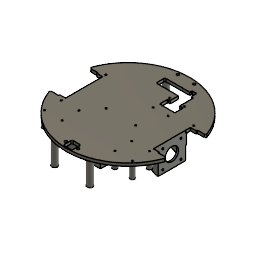
FEKTBOT_base_ver_1_2 (Autodesk Fusion 360 design; units mm, degrees)
Autodesk Fusion 360 part; units mm, degrees
note: some values were not read from the file. Set by a fixed rule: which sketch regions a step uses.
(part 1 of 2)
sketch "zakladna" plane through (0, 0, 0) normal (0, 1, 0) x (1, 0, 0)
  line L0 (-40.0372, -23.4927) -> (-85, -23.4927)
  line L1 (39.9628, -23.4927) -> (85, -23.4927)
  line L2 (-85, 23.5073) -> (-40.0372, 23.5073)
  line L3 (85, 23.5073) -> (39.9628, 23.5073)
  line L4 (1.75, 0) -> (22.5, 0)
  line L5 (-96.7123, 33.4364) -> (-85, 33.4364)
  line L6 (-85, 33.4364) -> (-85, 23.5073)
  line L7 (-96.7154, -33.4277) -> (-85, -33.4277)
  line L8 (-85, -33.4277) -> (-85, -23.4927)
  line L9 (96.7154, -33.4277) -> (85, -33.4277)
  line L10 (85, -33.4277) -> (85, -23.4927)
  line L11 (96.7123, 33.4364) -> (85, 33.4364)
  line L12 (85, 33.4364) -> (85, 23.5073)
  arc A0 (-98.5934, -36.1156) -> (98.5934, -36.1156) centre (0, 0) ccw
  arc A1 (-96.7154, -33.4277) -> (-98.5934, -36.1156) centre (-96.7154, -35.4277) ccw
  arc A2 (-98.5902, 36.1245) -> (-96.7123, 33.4364) centre (-96.7123, 35.4364) ccw
  arc A3 (96.7123, 33.4364) -> (98.5902, 36.1245) centre (96.7123, 35.4364) ccw
  arc A4 (98.5934, -36.1156) -> (96.7154, -33.4277) centre (96.7154, -35.4277) ccw
  line L13 (0, -1.75) -> (0, -22.5)
  line L14 (39.9628, -23.4927) -> (34.9628, -23.4927)
  line L15 (34.9628, -23.4927) -> (34.9628, 23.5073)
  line L16 (34.9628, 23.5073) -> (39.9628, 23.5073)
  line L17 (-40.0372, -23.4927) -> (-35.0372, -23.4927)
  line L18 (-35.0372, -23.4927) -> (-35.0372, 23.5073)
  line L19 (-35.0372, 23.5073) -> (-40.0372, 23.5073)
  line L20 (0, -20) -> (0, -2.5)
  line L21 (2.5, 0) -> (20, 0)
  line L22 (0, 105) -> (0, -105) construction
  line L23 (-105, 0) -> (104.2756, 0.0073) construction
  line L24 (-40, -12.9977) -> (44.2998, -12.9948) construction
  circle A5 centre (-25, -11.9963) radius 1.4
  circle A6 centre (-75, 37.0037) radius 1.4
  circle A7 centre (25, -11.9963) radius 1.4
  circle A8 centre (75, 37.0037) radius 1.4
  line L25 (-20, 83.0037) -> (20, 83.0037)
  line L26 (20, 83.0037) -> (20, 68.0037)
  line L27 (20, 68.0037) -> (-20, 68.0037)
  line L28 (-20, 68.0037) -> (-20, 83.0037)
  circle A9 centre (-10.5, -95.4967) radius 2.1
  circle A10 centre (10.5, -95.4967) radius 2.1
  line L29 (-5.5, -87.9967) -> (5.5, -87.9967)
  line L30 (7.5, -89.9967) -> (7.5, -100.9967)
  line L31 (5.5, -102.9967) -> (-5.5, -102.9967)
  line L32 (-7.5, -100.9967) -> (-7.5, -89.9967)
  line L33 (-10.5, -95.4967) -> (10.5, -95.4967) construction
  arc A11 (-5.5, -87.9967) -> (-7.5, -89.9967) centre (-5.5, -89.9967) ccw
  arc A12 (7.5, -89.9967) -> (5.5, -87.9967) centre (5.5, -89.9967) ccw
  arc A13 (5.5, -102.9967) -> (7.5, -100.9967) centre (5.5, -100.9967) ccw
  arc A14 (-7.5, -100.9967) -> (-5.5, -102.9967) centre (-5.5, -100.9967) ccw
  arc A15 (98.5902, 36.1245) -> (15, 103.923) centre (0, 0) ccw
  arc A16 (-15, 103.923) -> (-98.5902, 36.1245) centre (0, 0) ccw
  line L34 (75, -38.4927) -> (45, -38.4927) construction
  line L35 (45, -38.4927) -> (45, -67.4927) construction
  line L36 (45, -67.4927) -> (75, -67.4927) construction
  line L37 (75, -67.4927) -> (75, -38.4927) construction
  circle A17 centre (45, -38.4927) radius 1.375
  circle A18 centre (75, -38.4927) radius 1.375
  circle A19 centre (45, -67.4927) radius 1.375
  circle A20 centre (75, -67.4927) radius 1.375
  circle A21 centre (-45, -38.4927) radius 1.375
  circle A22 centre (-75, -38.4927) radius 1.375
  circle A23 centre (-75, -67.4927) radius 1.375
  circle A24 centre (-45, -67.4927) radius 1.375
  line L38 (34.9628, -23.4927) -> (74.9628, -23.4927)
  line L39 (74.9628, -23.4927) -> (74.9628, 23.5073)
  line L40 (74.9628, 23.5073) -> (34.9628, 23.5073)
  line L41 (34.9628, 23.5073) -> (34.9628, -23.4927)
  line L42 (-35.0372, -23.4927) -> (-75.0372, -23.4927)
  line L43 (-75.0372, -23.4927) -> (-75.0372, 23.5073)
  line L44 (-75.0372, 23.5073) -> (-35.0372, 23.5073)
  line L45 (-35.0372, 23.5073) -> (-35.0372, -23.4927)
  arc A25 (15, 103.923) -> (-15, 103.923) centre (0, 0) ccw
  line L46 (22, 99) -> (-25, 99) construction
  circle A26 centre (-14, 99) radius 2.1
  circle A27 centre (14, 99) radius 2.1
  point P0 (-82.0372, 22.8073)
  point P1 (-17.0372, -22.7927)
  point P2 (-0.0372, 0.0073)
  point P3 (81.9628, 22.8073)
  point P4 (-82.0372, -22.7927)
  point P5 (16.9628, 22.8073)
  point P6 (16.9628, 27.0073)
  point P7 (-17.0372, 27.0073)
  point P8 (81.9628, -22.7927)
  point P9 (16.9628, -22.7927)
  point P10 (16.9628, -26.9927)
  point P11 (-7.5, -87.9967)
  point P12 (7.5, -87.9967)
  point P13 (-7.5, -102.9967)
  dimension "d87" = 210
  dimension "d134" = 2
  dimension "d135" = 2
  dimension "d136" = 2
  dimension "d137" = 2
  dimension "d197" = 47
  dimension "d199" = 47
  dimension "d205" = 13
  dimension "d206" = 2.8
  dimension "d207" = 2.8
  dimension "d208" = 49
  dimension "d209" = 50
  dimension "d210" = 40
  dimension "d211" = 15
  dimension "d212" = 80
  dimension "d216" = 4.2
  dimension "d217" = 10.5
  dimension "d220" = 15
  dimension "d221" = 15
  dimension "d222" = 2
  dimension "d223" = 2
  dimension "d224" = 2
  dimension "d225" = 2
  dimension "d232" = 95.5
  dimension "d237" = 25
  dimension "d258" = 30
  dimension "d259" = 29
  dimension "d260" = 2.75
  dimension "d261" = 2.75
  dimension "d262" = 2.75
  dimension "d263" = 2.75
  dimension "d264" = 45
  dimension "d265" = 15
  dimension "d266" = 40
  dimension "d267" = 40
  dimension "d268" = 47
  dimension "d346" = 4.2
  dimension "d349" = 14
  constraint horizontal L2
  constraint horizontal L0
  constraint horizontal L3
  constraint horizontal L1
  constraint horizontal L5
  constraint vertical L6
  constraint horizontal L7
  constraint vertical L8
  constraint horizontal L9
  constraint vertical L10
  constraint horizontal L11
  constraint vertical L12
  constraint coincident A0.centre A15.centre
  constraint concentric A0 A15
  constraint tangent A0 A1
  constraint tangent L7 A1
  constraint tangent A2 A15
  constraint tangent L5 A2
  constraint tangent L11 A3
  constraint tangent A3 A15
  constraint tangent L9 A4
  constraint tangent A0 A4
  constraint horizontal L14
  constraint vertical L15
  constraint horizontal L16
  constraint horizontal L17
  constraint vertical L18
  constraint horizontal L19
  constraint midpoint A0 L22.end
  constraint parallel L20 L22
  constraint parallel L23 L24
  constraint symmetric L22 A5 A7
  constraint symmetric L22 A6 A8
  constraint horizontal L25
  constraint vertical L26
  constraint horizontal L27
  constraint vertical L28
  constraint symmetric L22 L26 L28
  constraint symmetric L22 A9 A10
  constraint horizontal L29
  constraint vertical L30
  constraint horizontal L31
  constraint vertical L32
  constraint symmetric L22 L30 L32
  constraint coincident A9.centre L33.start
  constraint coincident A10.centre L33.end
  constraint symmetric L29 L31 L33
  constraint coincident P11 L29
  constraint coincident P11 L32
  constraint tangent L29 A11
  constraint tangent L32 A11
  constraint coincident P12 L29
  constraint coincident P12 L30
  constraint tangent L29 A12
  constraint tangent L30 A12
  constraint tangent L30 A13
  constraint tangent L31 A13
  constraint coincident P13 L31
  constraint coincident P13 L32
  constraint tangent L31 A14
  constraint tangent L32 A14
  constraint concentric A15 A16
  constraint coincident L22.start A15
  constraint horizontal L34
  constraint vertical L35
  constraint horizontal L36
  constraint vertical L37
  constraint coincident L34.end L35.start
  constraint coincident L34.start L37.end
  constraint coincident L35.end L36.start
  constraint coincident L36.end L37.start
  constraint symmetric L22 A17 A21
  constraint symmetric L22 A18 A22
  constraint symmetric L22 A19 A24
  constraint symmetric L22 A20 A23
  constraint horizontal L38
  constraint vertical L39
  constraint horizontal L40
  constraint vertical L41
  constraint horizontal L42
  constraint vertical L43
  constraint horizontal L44
  constraint vertical L45
  constraint coincident L22.start A25
  constraint horizontal L46
  constraint coincident L46 A26.centre
  constraint symmetric L22 A26 A27
  measures "d87" diameter of A15
  measures "d134" radius of A1
  measures "d135" radius of A2
  measures "d136" radius of A3
  measures "d137" radius of A4
  measures "d197" distance of L1.start L3.end
  measures "d199" distance of L0.start L2.end
  measures "d205" distance of L23 L24
  measures "d206" diameter of A5
  measures "d207" diameter of A6
  measures "d208" vertical distance of A5.centre A6.centre
  measures "d209" horizontal distance of A5.centre A6.centre
  measures "d210" distance of L25.start L25.end
  measures "d211" distance of L25.start L27.end
  measures "d212" distance of A7.centre L27
  measures "d216" diameter of A9
  measures "d217" distance of L22 A9.centre
  measures "d220" distance of P11 P12
  measures "d221" distance of P11 P13
  measures "d222" radius of A11
  measures "d223" radius of A12
  measures "d224" radius of A13
  measures "d225" radius of A14
  measures "d232" distance of L23 A9.centre
  measures "d237" distance of L22 A5.centre
  measures "d258" distance of L34.start L34.end
  measures "d259" distance of L34.start L36.end
  measures "d260" diameter of A17
  measures "d261" diameter of A18
  measures "d262" diameter of A19
  measures "d263" diameter of A20
  measures "d264" distance of L22 L34.end
  measures "d265" distance of L1 L34.end
  measures "d266" distance of L14.end L38.end
  measures "d267" distance of L17.end L42.end
  measures "d268" distance of L17.end L18.end
  measures "d346" diameter of A26
  measures "d349" distance of L22 A26.centre
extrude "Extrude23" add sketch "zakladna" along normal blind 5 contours L0 L1 L2 L3 L5 L6 L7 L8 L9 L10 L11 L12 A0 A1 A2 A3 A4 L14 L15 L16 L17 L18 L19 A15 A16 L38 L40 L41 L42 L44 L45 A25 | A26 | A27
sketch "beterka" plane through (0, 0, 0) normal (0, 1, 0) x (1, 0, 0)
  line L0 (-34, -25) -> (34, -25)
  line L1 (34, -25) -> (34, -81)
  line L2 (34, -81) -> (-34, -81)
  line L3 (-34, -81) -> (-34, -25)
  line L4 (0, 105) -> (0, -105)
  line L5 (2.5, 0) -> (20, 0)
  line L6 (37.5, -84.5) -> (-37.5, -84.5)
  line L7 (-37.5, -84.5) -> (-37.5, -21.5)
  line L8 (-37.5, -21.5) -> (37.5, -21.5)
  line L9 (37.5, -21.5) -> (37.5, -84.5)
  dimension "d228" = 68
  dimension "d229" = 56
  dimension "d230" = 25
  dimension "d231" = -3.5
  constraint horizontal L0
  constraint vertical L1
  constraint horizontal L2
  constraint vertical L3
  constraint symmetric L1 L3 L4
  measures "d228" distance of L0.start L0.end
  measures "d229" distance of L0.start L2.end
  measures "d230" distance of L0 L5
extrude "Extrude25" add sketch "beterka" against normal blind 17 contours L0 L2 L3 L4 L6 L7 L8 | L0 L1 L2 L4 L6 L8 L9
sketch "zvyseni" plane through (0, 0, 0) normal (0, 1, 0) x (1, 0, 0)
  circle A0 centre (25, -11.9963) radius 4
  circle A1 centre (25, -11.9963) radius 1.4
  circle A2 centre (-25, -11.9963) radius 1.4
  circle A3 centre (-25, -11.9963) radius 4
  circle A4 centre (75, 37.0037) radius 1.4
  circle A5 centre (75, 37.0037) radius 4
  circle A6 centre (-75, 37.0037) radius 1.4
  circle A7 centre (-75, 37.0037) radius 4
  line L0 (5, 90) -> (-5, 90)
  line L1 (-5, 90) -> (-5, 85)
  line L2 (-5, 85) -> (5, 85)
  line L3 (5, 85) -> (5, 90)
  point P0 (25, -11.9963)
  point P1 (-25, -11.9963)
  point P2 (75, 37.0037)
  point P3 (-75, 37.0037)
  dimension "d250" = 8
  dimension "d251" = 8
  dimension "d252" = 8
  dimension "d253" = 8
  constraint coincident P0 A0.centre
  constraint coincident P1 A2.centre
  constraint coincident P2 A4.centre
  constraint concentric A4 A5
  constraint coincident P3 A6.centre
  constraint concentric A6 A7
  constraint horizontal L0
  constraint vertical L1
  constraint horizontal L2
  constraint vertical L3
  measures "d250" diameter of A0
  measures "d251" diameter of A3
  measures "d252" diameter of A5
  measures "d253" diameter of A7
extrude "Extrude26" add sketch "zvyseni" against normal blind 1.6
sketch " motory_podklad" plane through (0, 5, 0) normal (0, 1, 0) x (-1, 0, 0)
  circle A0 centre (-45, 67.4927) radius 1.375
  circle A1 centre (-10.5, 95.4967) radius 2.1
  circle A2 centre (-75, 38.4927) radius 1.375
  arc A3 (5.5, 87.9967) -> (7.5, 89.9967) centre (5.5, 89.9967) ccw
  line L0 (5.5, 87.9967) -> (-5.5, 87.9967)
  arc A4 (-7.5, 89.9967) -> (-5.5, 87.9967) centre (-5.5, 89.9967) ccw
  line L1 (-7.5, 89.9967) -> (-7.5, 100.9967)
  arc A5 (-5.5, 102.9967) -> (-7.5, 100.9967) centre (-5.5, 100.9967) ccw
  line L2 (-5.5, 102.9967) -> (5.5, 102.9967)
  arc A6 (7.5, 100.9967) -> (5.5, 102.9967) centre (5.5, 100.9967) ccw
  line L3 (7.5, 100.9967) -> (7.5, 89.9967)
  circle A7 centre (-75, -37.0037) radius 1.4
  circle A8 centre (25, 11.9963) radius 1.4
  circle A9 centre (-45, 38.4927) radius 1.375
  circle A10 centre (45, 67.4927) radius 1.375
  circle A11 centre (75, -37.0037) radius 1.4
  circle A12 centre (75, 67.4927) radius 1.375
  line L4 (-20, -68.0037) -> (20, -68.0037)
  line L5 (20, -68.0037) -> (20, -83.0037)
  line L6 (20, -83.0037) -> (-20, -83.0037)
  line L7 (-20, -83.0037) -> (-20, -68.0037)
  circle A13 centre (10.5, 95.4967) radius 2.1
  circle A14 centre (45, 38.4927) radius 1.375
  circle A15 centre (75, 38.4927) radius 1.375
  circle A16 centre (-25, 11.9963) radius 1.4
  circle A17 centre (-75, 67.4927) radius 1.375
  arc A18 (-96.7123, -33.4364) -> (-98.5902, -36.1245) centre (-96.7123, -35.4364) ccw
  arc A19 (-98.5902, -36.1245) -> (98.5902, -36.1245) centre (0, 0) ccw
  arc A20 (98.5902, -36.1245) -> (96.7123, -33.4364) centre (96.7123, -35.4364) ccw
  line L8 (96.7123, -33.4364) -> (85, -33.4364)
  line L9 (85, -33.4364) -> (85, -23.5073)
  line L10 (85, -23.5073) -> (35.0372, -23.5073)
  line L11 (35.0372, -23.5073) -> (35.0372, 23.4927)
  line L12 (35.0372, 23.4927) -> (85, 23.4927)
  line L13 (85, 23.4927) -> (85, 33.4277)
  line L14 (85, 33.4277) -> (96.7154, 33.4277)
  arc A21 (96.7154, 33.4277) -> (98.5934, 36.1156) centre (96.7154, 35.4277) ccw
  arc A22 (98.5934, 36.1156) -> (-98.5934, 36.1156) centre (0, 0) ccw
  arc A23 (-98.5934, 36.1156) -> (-96.7154, 33.4277) centre (-96.7154, 35.4277) ccw
  line L15 (-96.7154, 33.4277) -> (-85, 33.4277)
  line L16 (-85, 33.4277) -> (-85, 23.4927)
  line L17 (-85, 23.4927) -> (-34.9628, 23.4927)
  line L18 (-34.9628, 23.4927) -> (-34.9628, -23.5073)
  line L19 (-34.9628, -23.5073) -> (-85, -23.5073)
  line L20 (-85, -23.5073) -> (-85, -33.4364)
  line L21 (-85, -33.4364) -> (-96.7123, -33.4364)
  line L22 (75.0372, -23.5073) -> (35.0372, -23.5073)
  line L23 (35.0372, -23.5073) -> (35.0372, 23.4927)
  line L24 (35.0372, 23.4927) -> (75.0372, 23.4927)
  line L25 (75.0372, 23.4927) -> (75.0372, -23.5073)
  line L26 (-34.9628, -23.5073) -> (-74.9628, -23.5073)
  line L27 (-74.9628, -23.5073) -> (-74.9628, 23.4927)
  line L28 (-74.9628, 23.4927) -> (-34.9628, 23.4927)
  line L29 (-34.9628, 23.4927) -> (-34.9628, -23.5073)
  line L30 (75.0372, 23.4927) -> (75.0372, -23.5073)
  line L31 (35.0372, 23.4927) -> (75.0372, 23.4927)
  point P0 (75.0372, -23.5073)
  point P1 (-74.9628, 23.4927)
  dimension "d271" = 47
  dimension "d272" = 40
  constraint horizontal L22
  constraint vertical L23
  constraint horizontal L24
  constraint vertical L25
  constraint coincident L11.end L12.start
  constraint coincident P0 L22.start
  constraint horizontal L26
  constraint vertical L27
  constraint horizontal L28
  constraint vertical L29
  constraint coincident P1 L27.end
  constraint coincident L18.end L19.start
  measures "d271" distance of L24.end P0
  measures "d272" distance of L24.end L11.end
extrude "Extrude27" add sketch " motory_podklad" against normal blind 45 contours L17 L18 L19 L26 L27 L28 L29 | L10 L11 L12 L22 L23 L24 L25 L30 L31
sketch "motory_kapsa" plane through (0, -40, 0) normal (0, -1, 0) x (1, 0, 0)
  line L0 (-35.0372, 23.4927) -> (-75.0372, 23.4927)
  line L1 (-75.0372, 23.4927) -> (-75.0372, -23.5073)
  line L2 (-75.0372, -23.5073) -> (-35.0372, -23.5073)
  line L3 (-35.0372, -23.5073) -> (-35.0372, 23.4927)
  line L4 (-35.0372, 21.4927) -> (-72.0372, 21.4927)
  line L5 (-72.0372, 21.4927) -> (-72.0372, -21.5073)
  line L6 (-72.0372, -21.5073) -> (-35.0372, -21.5073)
  line L7 (-35.0372, -21.5073) -> (-35.0372, 21.4927)
  line L8 (0, -105) -> (0, 105)
  line L9 (34.9628, 21.4927) -> (71.9628, 21.4927)
  line L10 (71.9628, 21.4927) -> (71.9628, -21.5073)
  line L11 (71.9628, -21.5073) -> (34.9628, -21.5073)
  line L12 (34.9628, -21.5073) -> (34.9628, 21.4927)
  line L13 (34.9628, -23.5073) -> (34.9628, 23.4927)
  line L14 (74.9628, 23.4927) -> (34.9628, 23.4927)
  dimension "d273" = 37
  dimension "d274" = 43
  dimension "d275" = 2
  dimension "d278" = 37
  dimension "d279" = 43
  dimension "d280" = 2
  constraint horizontal L4
  constraint vertical L5
  constraint horizontal L6
  constraint vertical L7
  constraint coincident L3 L4.start
  constraint horizontal L9
  constraint vertical L10
  constraint horizontal L11
  constraint vertical L12
  constraint coincident L9.start L13
  measures "d273" distance of L4.start L4.end
  measures "d274" distance of L4.start L6.end
  measures "d275" distance of L0 L4
  measures "d278" distance of L9.start L9.end
  measures "d279" distance of L9.start L11.end
  measures "d280" distance of L9 L14
extrude "Extrude29" cut sketch "motory_kapsa" against normal blind 43 contours L3 L4 L5 L6 L7 | L9 L10 L11 L12 L13
sketch "motory_diry" plane through (71.9628, 0, 0) normal (-1, 0, 0) x (0, 0, 1)
  line L0 (-21.5073, -40) -> (21.4927, -40)
  line L1 (21.4927, -40) -> (21.4927, 3)
  line L2 (21.4927, 3) -> (-21.5073, 3)
  line L3 (-21.5073, 3) -> (-21.5073, -40)
  line L4 (0, -26.6328) -> (0, -8.6328) construction
  line L5 (23, -18.5) -> (-28, -18.5) construction
  circle A0 centre (0, -18.5) radius 11.25
  circle A1 centre (15.5, -34) radius 1.6
  circle A2 centre (-15.5, -34) radius 1.6
  circle A3 centre (15.5, -3) radius 1.6
  circle A4 centre (-15.5, -3) radius 1.6
  dimension "d283" = 43
  dimension "d284" = 43
  dimension "d285" = 21.5
  dimension "d286" = 22.5
  dimension "d287" = 3.2
  dimension "d288" = 15.5
  dimension "d289" = 15.5
  constraint vertical L4
  constraint perpendicular L3 L5
  constraint coincident L4 A0.centre
  constraint coincident L5 A0.centre
  constraint symmetric L4 A1 A2
  constraint symmetric L5 A1 A3
  constraint symmetric L5 A2 A4
  measures "d283" distance of L0.end L1.end
  measures "d284" distance of L0.start L0.end
  measures "d285" distance of L2 L5
  measures "d286" diameter of A0
  measures "d287" diameter of A1
  measures "d288" distance of L4 A1.centre
  measures "d289" distance of L5 A1.centre
extrude "Extrude30" cut sketch "motory_diry" along normal through all and the other way through all contours A0 | A1 | A2 | A3 | A4
sketch "Sketch20" plane through (0, 0, 23.4927) normal (0, 0, 1) x (1, 0, 0)
  line L0 (74.9628, 0) -> (37.5, 0)
  line L1 (34.9628, -17) -> (34.9628, -40)
  line L2 (34.9628, -40) -> (74.9628, -40)
  line L3 (74.9628, -40) -> (74.9628, 0)
  line L4 (71.9628, -40) -> (39.9159, -25.4626)
  line L5 (39.9159, -25.4626) -> (39.9159, -17)
  line L6 (37.5, -17) -> (-37.5, -17)
  line L7 (39.9159, -17) -> (0, -17)
  line L8 (0, -40) -> (71.9628, -40)
  line L9 (0, 2.5) -> (0, 20)
  line L10 (-71.9628, -40) -> (-39.9159, -25.4626)
  line L11 (0, -40) -> (-71.9628, -40)
  line L12 (-39.9159, -25.4626) -> (-39.9159, -17)
  line L13 (-39.9159, -17) -> (0, -17)
  line L14 (37.5, 0) -> (37.5, -17)
  line L15 (37.5, -17) -> (34.9628, -17)
  point P0 (71.9628, -40)
  point P1 (71.9628, -40)
  constraint coincident P1 P0
  constraint perpendicular L2 L5
  constraint midpoint L6 L7.end
  constraint symmetric P1 L9 L10.start
  constraint symmetric L4.end L9 L10.end
  constraint symmetric L5.end L9 L12.end
  constraint symmetric L7.end L9 L13.end
  constraint symmetric L8.start L9 L11.start
extrude "Extrude32" cut sketch "Sketch20" against normal blind 53 contours L1 L2 L4 L5 L6 L7 L8 L15 | L1 L6 L7 L8 L10 L11 L12 L13
chamfer "Chamfer1" distance 3 angle 45 2 edges at (34.9628, 0, -0.0073) (-35.0372, 0, -0.0073)
sketch "Drzaky_displeje" plane through (0, 0, 0) normal (0, -1, 0) x (1, 0, 0)
  line L0 (34.9628, 21.5) -> (-35.0372, 21.5)
  line L1 (-20, -68.0037) -> (20, -68.0037)
  line L2 (20, -68.0037) -> (20, -83.0037)
  line L3 (20, -83.0037) -> (-20, -83.0037)
  line L4 (-20, -83.0037) -> (-20, -68.0037)
  circle A0 centre (-25, 11.9963) radius 4
  circle A1 centre (75, -37.0037) radius 4
  circle A2 centre (25, 11.9963) radius 4
  circle A3 centre (-75, -37.0037) radius 4
  line L5 (5, -90) -> (-5, -90)
  line L6 (-5, -90) -> (-5, -85)
  line L7 (-5, -85) -> (5, -85)
  line L8 (5, -85) -> (5, -90)
  line L9 (-35.0372, 21.4927) -> (-32.0372, 21.4927)
  line L10 (-32.0372, 21.4927) -> (-32.0372, -21.5073)
  line L11 (-32.0372, -21.5073) -> (-35.0372, -21.5073)
  line L12 (-35.0372, -21.5073) -> (-35.0372, -23.5073)
  line L13 (-35.0372, -23.5073) -> (-75.0372, -23.5073)
  line L14 (-75.0372, -23.5073) -> (-85, -23.5073)
  line L15 (-85, -23.5073) -> (-85, -33.4364)
  line L16 (-85, -33.4364) -> (-96.7123, -33.4364)
  arc A4 (-96.7123, -33.4364) -> (-98.5902, -36.1245) centre (-96.7123, -35.4364) ccw
  arc A5 (-98.5902, -36.1245) -> (98.5902, -36.1245) centre (0, 0) ccw
  arc A6 (98.5902, -36.1245) -> (96.7123, -33.4364) centre (96.7123, -35.4364) ccw
  line L17 (96.7123, -33.4364) -> (85, -33.4364)
  line L18 (85, -33.4364) -> (85, -23.5073)
  line L19 (85, -23.5073) -> (74.9628, -23.5073)
  line L20 (74.9628, -23.5073) -> (34.9628, -23.5073)
  line L21 (34.9628, -23.5073) -> (34.9628, -21.5073)
  line L22 (34.9628, -21.5073) -> (31.9628, -21.5073)
  line L23 (31.9628, -21.5073) -> (31.9628, 21.4927)
  line L24 (31.9628, 21.4927) -> (34.9628, 21.4927)
  line L25 (34.9628, 21.4927) -> (34.9628, 21.5)
  line L26 (-35.0372, 21.5) -> (-35.0372, 21.4927)
  circle A7 centre (-75, 38.4927) radius 4
  circle A8 centre (-45, 38.4927) radius 4
  circle A9 centre (-45, 67.4927) radius 4
  circle A10 centre (-75, 67.4927) radius 4
  circle A11 centre (-75, 67.4927) radius 1.375
  circle A12 centre (-45, 67.4927) radius 1.375
  circle A13 centre (-45, 38.4927) radius 1.375
  circle A14 centre (-75, 38.4927) radius 1.375
  circle A15 centre (45, 67.4927) radius 4
  circle A16 centre (45, 38.4927) radius 4
  circle A17 centre (75, 38.4927) radius 4
  circle A18 centre (75, 67.4927) radius 4
  circle A19 centre (45, 38.4927) radius 1.375
  circle A20 centre (75, 38.4927) radius 1.375
  circle A21 centre (75, 67.4927) radius 1.375
  circle A22 centre (45, 67.4927) radius 1.375
  dimension "d300" = 8
  dimension "d301" = 8
  dimension "d302" = 8
  dimension "d303" = 8
  dimension "d304" = 8
  dimension "d305" = 8
  dimension "d306" = 8
  dimension "d307" = 8
  measures "d300" diameter of A7
  measures "d301" diameter of A8
  measures "d302" diameter of A9
  measures "d303" diameter of A10
  measures "d304" diameter of A15
  measures "d305" diameter of A16
  measures "d306" diameter of A17
  measures "d307" diameter of A18
extrude "Extrude33" add sketch "Drzaky_displeje" along normal blind 20 contours A7 | A8 | A9 | A10 | A15 | A16 | A17 | A18
fillet "Fillet4" radius 2 4 edges at (20, 2.5, -68.0037) (-20, 2.5, -68.0037) (20, 2.5, -83.0037) (-20, 2.5, -83.0037)
sketch "Sketch22" plane through (0, 0, 0) normal (0, -1, 0) x (1, 0, 0)
  line L0 (34.9628, 21.5) -> (-35.0372, 21.5)
  arc A0 (20, -70.0037) -> (18, -68.0037) centre (18, -70.0037) ccw
  line L1 (20, -70.0037) -> (20, -81.0037)
  arc A1 (18, -83.0037) -> (20, -81.0037) centre (18, -81.0037) ccw
  line L2 (18, -83.0037) -> (-18, -83.0037)
  arc A2 (-20, -81.0037) -> (-18, -83.0037) centre (-18, -81.0037) ccw
  line L3 (-20, -81.0037) -> (-20, -70.0037)
  arc A3 (-18, -68.0037) -> (-20, -70.0037) centre (-18, -70.0037) ccw
  line L4 (-18, -68.0037) -> (18, -68.0037)
  circle A4 centre (-25, 11.9963) radius 4
  circle A5 centre (75, -37.0037) radius 4
  circle A6 centre (25, 11.9963) radius 4
  circle A7 centre (-75, -37.0037) radius 4
  line L5 (5, -90) -> (-5, -90)
  line L6 (-5, -90) -> (-5, -85)
  line L7 (-5, -85) -> (5, -85)
  line L8 (5, -85) -> (5, -90)
  line L9 (-35.0372, 21.4927) -> (-32.0372, 21.4927)
  line L10 (-32.0372, 21.4927) -> (-32.0372, -21.5073)
  line L11 (-32.0372, -21.5073) -> (-35.0372, -21.5073)
  line L12 (-35.0372, -21.5073) -> (-35.0372, -23.5073)
  line L13 (-35.0372, -23.5073) -> (-75.0372, -23.5073)
  line L14 (-75.0372, -23.5073) -> (-85, -23.5073)
  line L15 (-85, -23.5073) -> (-85, -33.4364)
  line L16 (-85, -33.4364) -> (-96.7123, -33.4364)
  arc A8 (-96.7123, -33.4364) -> (-98.5902, -36.1245) centre (-96.7123, -35.4364) ccw
  arc A9 (-98.5902, -36.1245) -> (98.5902, -36.1245) centre (0, 0) ccw
  arc A10 (98.5902, -36.1245) -> (96.7123, -33.4364) centre (96.7123, -35.4364) ccw
  line L17 (96.7123, -33.4364) -> (85, -33.4364)
  line L18 (85, -33.4364) -> (85, -23.5073)
  line L19 (85, -23.5073) -> (74.9628, -23.5073)
  line L20 (74.9628, -23.5073) -> (34.9628, -23.5073)
  line L21 (34.9628, -23.5073) -> (34.9628, -21.5073)
  line L22 (34.9628, -21.5073) -> (31.9628, -21.5073)
  line L23 (31.9628, -21.5073) -> (31.9628, 21.4927)
  line L24 (31.9628, 21.4927) -> (34.9628, 21.4927)
  line L25 (34.9628, 21.4927) -> (34.9628, 21.5)
  line L26 (-35.0372, 21.5) -> (-35.0372, 21.4927)
  line L27 (74.9628, -23.5073) -> (34.9628, -23.5073)
  line L28 (34.9628, -23.5073) -> (34.9628, -25.0073)
  line L29 (34.9628, -25.0073) -> (74.9628, -25.0073)
  line L30 (74.9628, -25.0073) -> (74.9628, -23.5073)
  line L31 (74.9628, 23.4927) -> (37.5, 23.4927)
  line L32 (37.5, 23.4927) -> (37.5, 24.9927)
  line L33 (37.5, 24.9927) -> (74.9628, 24.9927)
  line L34 (74.9628, 24.9927) -> (74.9628, 23.4927)
  line L35 (0, 1.75) -> (0, 22.5)
  line L36 (-34.9628, -25.0073) -> (-74.9628, -25.0073)
  line L37 (-74.9628, -25.0073) -> (-74.9628, -23.5073)
  line L38 (-74.9628, -23.5073) -> (-34.9628, -23.5073)
  line L39 (-34.9628, -23.5073) -> (-34.9628, -25.0073)
  line L40 (-74.9628, 24.9927) -> (-74.9628, 23.4927)
  line L41 (-37.5, 24.9927) -> (-74.9628, 24.9927)
  line L42 (-74.9628, 23.4927) -> (-37.5, 23.4927)
  line L43 (-37.5, 23.4927) -> (-37.5, 24.9927)
  dimension "d312" = 1.5
  dimension "d313" = 1.5
  constraint horizontal L27
  constraint vertical L28
  constraint horizontal L29
  constraint vertical L30
  constraint coincident L19.end L20.start
  constraint horizontal L31
  constraint vertical L32
  constraint horizontal L33
  constraint vertical L34
  constraint symmetric L19.end L35 L37.end
  constraint symmetric L20.end L35 L38.end
  constraint symmetric L28.end L35 L36.start
  constraint symmetric L29.end L35 L36.end
  constraint symmetric L31.start L35 L40.end
  constraint symmetric L31.end L35 L42.end
  constraint symmetric L32.end L35 L41.start
  constraint symmetric L33.end L35 L40.start
  measures "d312" distance of L19.end L29.end
  measures "d313" distance of L31.start L33.end
extrude "Extrude34" add sketch "Sketch22" along normal blind 17 contours L20 L27 L28 L29 L30 | L13 L36 L37 L38 L39 | L31 L32 L33 L34 | L40 L41 L42 L43
fillet "Fillet5" radius 5 2 edges at (56.2314, 0, 24.9927) (-56.2314, 0, 24.9927)
fillet "Fillet6" radius 2 2 edges at (-54.9628, 0, -25.0073) (54.9628, 0, -25.0073)
fillet "Fillet7" radius 1.5 2 edges at (57.4394, -17, -23.5073) (57.4394, -17, 23.4927)
sketch "Sketch24" plane through (0, 5, 0) normal (0, 1, 0) x (-1, 0, 0)
  line L0 (-85, -23.5073) -> (-85, -33.4364)
  line L1 (-85, -33.4364) -> (-96.7123, -33.4364)
  arc A0 (-96.7123, -33.4364) -> (-98.5902, -36.1245) centre (-96.7123, -35.4364) ccw
  arc A1 (-98.5902, -36.1245) -> (98.5902, -36.1245) centre (0, 0) ccw
  arc A2 (98.5902, -36.1245) -> (96.7123, -33.4364) centre (96.7123, -35.4364) ccw
  line L2 (96.7123, -33.4364) -> (85, -33.4364)
  line L3 (85, -33.4364) -> (85, -23.5073)
  line L4 (75.0372, -23.5073) -> (75.0372, 23.4927)
  line L5 (85, 23.4927) -> (85, 33.4277)
  line L6 (85, 33.4277) -> (96.7154, 33.4277)
  arc A3 (96.7154, 33.4277) -> (98.5934, 36.1156) centre (96.7154, 35.4277) ccw
  arc A4 (98.5934, 36.1156) -> (-98.5934, 36.1156) centre (0, 0) ccw
  arc A5 (-98.5934, 36.1156) -> (-96.7154, 33.4277) centre (-96.7154, 35.4277) ccw
  line L7 (-96.7154, 33.4277) -> (-85, 33.4277)
  line L8 (-85, 33.4277) -> (-85, 23.4927)
  line L9 (-74.9628, 23.4927) -> (-74.9628, -23.5073)
  line L10 (-74.9628, -23.5073) -> (-85, -23.5073)
  circle A6 centre (75, 67.4927) radius 1.375
  circle A7 centre (-25, 11.9963) radius 1.4
  circle A8 centre (-10.5, 95.4967) radius 2.1
  circle A9 centre (-75, 67.4927) radius 1.375
  circle A10 centre (75, 38.4927) radius 1.375
  circle A11 centre (10.5, 95.4967) radius 2.1
  circle A12 centre (-45, 67.4927) radius 1.375
  circle A13 centre (-45, 38.4927) radius 1.375
  circle A14 centre (45, 38.4927) radius 1.375
  arc A15 (5.5, 87.9967) -> (7.5, 89.9967) centre (5.5, 89.9967) ccw
  line L11 (5.5, 87.9967) -> (-5.5, 87.9967)
  arc A16 (-7.5, 89.9967) -> (-5.5, 87.9967) centre (-5.5, 89.9967) ccw
  line L12 (-7.5, 89.9967) -> (-7.5, 100.9967)
  arc A17 (-5.5, 102.9967) -> (-7.5, 100.9967) centre (-5.5, 100.9967) ccw
  line L13 (-5.5, 102.9967) -> (5.5, 102.9967)
  arc A18 (7.5, 100.9967) -> (5.5, 102.9967) centre (5.5, 100.9967) ccw
  line L14 (7.5, 100.9967) -> (7.5, 89.9967)
  circle A19 centre (-75, 38.4927) radius 1.375
  line L15 (-18, -68.0037) -> (18, -68.0037)
  arc A20 (20, -70.0037) -> (18, -68.0037) centre (18, -70.0037) ccw
  line L16 (20, -70.0037) -> (20, -81.0037)
  arc A21 (18, -83.0037) -> (20, -81.0037) centre (18, -81.0037) ccw
  line L17 (18, -83.0037) -> (-18, -83.0037)
  arc A22 (-20, -81.0037) -> (-18, -83.0037) centre (-18, -81.0037) ccw
  line L18 (-20, -81.0037) -> (-20, -70.0037)
  arc A23 (-18, -68.0037) -> (-20, -70.0037) centre (-18, -70.0037) ccw
  circle A24 centre (75, -37.0037) radius 1.4
  circle A25 centre (25, 11.9963) radius 1.4
  circle A26 centre (45, 67.4927) radius 1.375
  circle A27 centre (-75, -37.0037) radius 1.4
  line L19 (85, -23.5073) -> (75.0372, -23.5073)
  line L20 (75.0372, 23.4927) -> (85, 23.4927)
  line L21 (-85, 23.4927) -> (-74.9628, 23.4927)
fillet "Fillet8" radius 1.5 2 edges at (-57.4394, -17, 23.4927) (-57.4394, -17, -23.5073)
sketch "RFID" plane through (0, 5, 0) normal (0, 1, 0) x (-1, 0, 0)
  circle A0 centre (75, 67.4927) radius 1.375
  circle A1 centre (-25, 11.9963) radius 1.4
  circle A2 centre (-10.5, 95.4967) radius 2.1
  circle A3 centre (-75, 67.4927) radius 1.375
  circle A4 centre (75, 38.4927) radius 1.375
  circle A5 centre (10.5, 95.4967) radius 2.1
  circle A6 centre (-45, 67.4927) radius 1.375
  circle A7 centre (-45, 38.4927) radius 1.375
  circle A8 centre (45, 38.4927) radius 1.375
  arc A9 (5.5, 87.9967) -> (7.5, 89.9967) centre (5.5, 89.9967) ccw
  line L0 (5.5, 87.9967) -> (-5.5, 87.9967)
  arc A10 (-7.5, 89.9967) -> (-5.5, 87.9967) centre (-5.5, 89.9967) ccw
  line L1 (-7.5, 89.9967) -> (-7.5, 100.9967)
  arc A11 (-5.5, 102.9967) -> (-7.5, 100.9967) centre (-5.5, 100.9967) ccw
  line L2 (-5.5, 102.9967) -> (5.5, 102.9967)
  arc A12 (7.5, 100.9967) -> (5.5, 102.9967) centre (5.5, 100.9967) ccw
  line L3 (7.5, 100.9967) -> (7.5, 89.9967)
  circle A13 centre (-75, 38.4927) radius 1.375
  line L4 (-18, -68.0037) -> (18, -68.0037)
  arc A14 (20, -70.0037) -> (18, -68.0037) centre (18, -70.0037) ccw
  line L5 (20, -70.0037) -> (20, -81.0037)
  arc A15 (18, -83.0037) -> (20, -81.0037) centre (18, -81.0037) ccw
  line L6 (18, -83.0037) -> (-18, -83.0037)
  arc A16 (-20, -81.0037) -> (-18, -83.0037) centre (-18, -81.0037) ccw
  line L7 (-20, -81.0037) -> (-20, -70.0037)
  arc A17 (-18, -68.0037) -> (-20, -70.0037) centre (-18, -70.0037) ccw
  circle A18 centre (75, -37.0037) radius 1.4
  circle A19 centre (25, 11.9963) radius 1.4
  circle A20 centre (45, 67.4927) radius 1.375
  circle A21 centre (-75, -37.0037) radius 1.4
  arc A22 (-96.7123, -33.4364) -> (-98.5902, -36.1245) centre (-96.7123, -35.4364) ccw
  arc A23 (-98.5902, -36.1245) -> (98.5902, -36.1245) centre (0, 0) ccw
  arc A24 (98.5902, -36.1245) -> (96.7123, -33.4364) centre (96.7123, -35.4364) ccw
  line L8 (96.7123, -33.4364) -> (85, -33.4364)
  line L9 (85, -33.4364) -> (85, -23.5073)
  line L10 (85, -23.5073) -> (75.0372, -23.5073)
  line L11 (75.0372, -23.5073) -> (75.0372, 23.4927)
  line L12 (75.0372, 23.4927) -> (85, 23.4927)
  line L13 (85, 23.4927) -> (85, 33.4277)
  line L14 (85, 33.4277) -> (96.7154, 33.4277)
  arc A25 (96.7154, 33.4277) -> (98.5934, 36.1156) centre (96.7154, 35.4277) ccw
  arc A26 (98.5934, 36.1156) -> (-98.5934, 36.1156) centre (0, 0) ccw
  arc A27 (-98.5934, 36.1156) -> (-96.7154, 33.4277) centre (-96.7154, 35.4277) ccw
  line L15 (-96.7154, 33.4277) -> (-85, 33.4277)
  line L16 (-85, 33.4277) -> (-85, 23.4927)
  line L17 (-85, 23.4927) -> (-74.9628, 23.4927)
  line L18 (-74.9628, 23.4927) -> (-74.9628, -23.5073)
  line L19 (-74.9628, -23.5073) -> (-85, -23.5073)
  line L20 (-85, -23.5073) -> (-85, -33.4364)
  line L21 (-85, -33.4364) -> (-96.7123, -33.4364)
  line L22 (-46.4, -22) -> (-6, -22) construction
  line L23 (-6, -22) -> (-6, -64.7) construction
  line L24 (-6, -64.7) -> (-46.4, -64.7) construction
  line L25 (-46.4, -64.7) -> (-46.4, -22) construction
  line L26 (0, -105) -> (0, 105) construction
  line L27 (-2.5, 0) -> (-20, 0) construction
  line L28 (-38.8, -29.45) -> (-13.6, -29.45) construction
  line L29 (-13.6, -29.45) -> (-13.6, -57.25) construction
  line L30 (-13.6, -57.25) -> (-38.8, -57.25) construction
  line L31 (-38.8, -57.25) -> (-38.8, -29.45) construction
  line L32 (-39.9159, 23.4927) -> (-74.9628, 23.4927) construction
  line L33 (-26.2, -7.8505) -> (-26.2, -73.1555) construction
  line L34 (-55, -43.35) -> (-4, -43.35) construction
  circle A28 centre (-38.8, -29.45) radius 1.35
  circle A29 centre (-13.6, -29.45) radius 1.35
  circle A30 centre (-38.8, -57.25) radius 1.35
  circle A31 centre (-13.6, -57.25) radius 1.35
  line L35 (-23, -73) -> (-29, -73)
  line L36 (-30, -74) -> (-30, -86)
  line L37 (-29, -87) -> (-23, -87)
  line L38 (-22, -86) -> (-22, -74)
  arc A32 (-29, -73) -> (-30, -74) centre (-29, -74) ccw
  arc A33 (-22, -74) -> (-23, -73) centre (-23, -74) ccw
  arc A34 (-30, -86) -> (-29, -87) centre (-29, -86) ccw
  arc A35 (-23, -87) -> (-22, -86) centre (-23, -86) ccw
  line L39 (-85, -23.5073) -> (-75, -23.5073)
  line L40 (-75, -23.5073) -> (-75, -31.5073)
  line L41 (-75, -31.5073) -> (-85, -31.5073)
  line L42 (-85, -31.5073) -> (-85, -23.5073)
  line L43 (-85, 23.4927) -> (-74.9628, 23.4927)
  line L44 (-74.9628, 23.4927) -> (-74.9628, 31.4927)
  line L45 (-74.9628, 31.4927) -> (-85, 31.4927)
  line L46 (-85, 31.4927) -> (-85, 23.4927)
  line L47 (85, 23.4927) -> (74.9628, 23.4927)
  line L48 (74.9628, 23.4927) -> (74.9628, 31.4927)
  line L49 (74.9628, 31.4927) -> (85, 31.4927)
  line L50 (85, 31.4927) -> (85, 23.4927)
  line L51 (85, -23.5073) -> (75, -23.5073)
  line L52 (75, -23.5073) -> (75, -31.5073)
  line L53 (75, -31.5073) -> (85, -31.5073)
  line L54 (85, -31.5073) -> (85, -23.5073)
  dimension "d324" = 40.4
  dimension "d325" = 42.7
  dimension "d326" = 6
  dimension "d327" = 22
  dimension "d328" = 25.2
  dimension "d329" = 27.8
  dimension "d330" = 26.2
  dimension "d331" = 43.35
  dimension "d332" = 2.7
  dimension "d333" = 2.7
  dimension "d334" = 2.7
  dimension "d335" = 2.7
  dimension "d336" = 1
  dimension "d337" = 1
  dimension "d338" = 1
  dimension "d339" = 1
  dimension "d340" = 8
  dimension "d341" = 8
  dimension "d342" = 8
  dimension "d343" = 8
  constraint horizontal L22
  constraint vertical L23
  constraint horizontal L24
  constraint vertical L25
  constraint horizontal L28
  constraint vertical L29
  constraint horizontal L30
  constraint vertical L31
  constraint perpendicular L32 L33
  constraint symmetric L29 L31 L33
  constraint perpendicular L23 L34
  constraint symmetric L28 L30 L34
  constraint coincident L28.start L31.end
  constraint coincident L28.end L29.start
  constraint coincident L30.end L31.start
  constraint coincident L29.end L30.start
  constraint horizontal L35
  constraint vertical L36
  constraint horizontal L37
  constraint vertical L38
  constraint tangent L35 A32
  constraint tangent L36 A32
  constraint tangent L35 A33
  constraint tangent L38 A33
  constraint tangent L36 A34
  constraint tangent L37 A34
  constraint tangent L37 A35
  constraint tangent L38 A35
  constraint horizontal L39
  constraint vertical L40
  constraint horizontal L41
  constraint vertical L42
  constraint coincident L19.end L20.start
  constraint horizontal L43
  constraint vertical L44
  constraint horizontal L45
  constraint vertical L46
  constraint coincident L16.end L17.start
  constraint horizontal L47
  constraint vertical L48
  constraint horizontal L49
  constraint vertical L50
  constraint coincident L12.end L13.start
  constraint horizontal L51
  constraint vertical L52
  constraint horizontal L53
  constraint vertical L54
  constraint coincident L9.end L10.start
  measures "d324" distance of L22.start L22.end
  measures "d325" distance of L22.start L24.end
  measures "d326" distance of L23 L26
  measures "d327" distance of L22 L27
  measures "d328" distance of L28.start L28.end
  measures "d329" distance of L28.start L30.end
  measures "d330" distance of L26 L33
  measures "d331" distance of L27 L34
  measures "d332" diameter of A28
  measures "d333" diameter of A29
  measures "d334" diameter of A30
  measures "d335" diameter of A31
  measures "d336" radius of A32
  measures "d337" radius of A33
  measures "d338" radius of A34
  measures "d339" radius of A35
  measures "d340" distance of L19.end L41.end
  measures "d341" distance of L16.end L45.end
  measures "d342" distance of L12.end L49.end
  measures "d343" distance of L9.end L53.end
extrude "Extrude35" cut sketch "RFID" against normal blind 5 contours L19 L20 L39 L40 L41 L42 | L9 L10 L51 L52 L53 L54 | L16 L17 L43 L44 L45 L46 | L12 L13 L47 L48 L49 L50 | A28 | A29 | A30 | A31 | L35 L36 L37 L38 A32 A33 A34 A35
extrude "Extrude36" cut sketch "zakladna" along normal blind 5 contours A26 | A27
sketch "VL53" plane through (0, 0, 0) normal (0, 1, 0) x (1, 0, 0)
  line L0 (-7.75, 101) -> (7.75, 101)
  line L1 (7.75, 101) -> (7.75, 102.7)
  line L2 (7.75, 102.7) -> (-7.75, 102.7)
  line L3 (-7.75, 102.7) -> (-7.75, 101)
  line L4 (0, 105) -> (0, -105)
  line L5 (9.45, 104.4) -> (-9.45, 104.4)
  line L6 (-9.45, 104.4) -> (-9.45, 99.3)
  line L7 (-9.45, 99.3) -> (9.45, 99.3)
  line L8 (9.45, 99.3) -> (9.45, 104.4)
  dimension "d350" = 15.5
  dimension "d351" = 1.7
  dimension "d352" = 1.7
  constraint horizontal L0
  constraint vertical L1
  constraint horizontal L2
  constraint vertical L3
  constraint symmetric L1 L3 L4
  measures "d350" distance of L0.start L0.end
  measures "d351" distance of L0.start L2.end
  measures "d352" distance of L1
extrude "Extrude37" add sketch "VL53" against normal blind 5.6 contours L0 L2 L3 L4 L5 L6 L7
extrude "Extrude38" add sketch "VL53" against normal blind 5.6 contours L0 L1 L2 L4 L5 L7 L8
fillet "Fillet9" radius 0.5 8 edges at (-9.45, -2.8, -104.4) (9.45, -2.8, -104.4) (9.45, -2.8, -99.3) (-9.45, -2.8, -99.3) (-9.45, -5.6, -101.85) (0, -5.6, -104.4) (9.45, -5.6, -101.85) (0, -5.6, -99.3)
fillet "Fillet10" radius 0.5 8 edges at (9.3036, 0, -99.4464) (9.45, 0, -101.85) (9.3036, 0, -104.2536) (0, 0, -104.4) (-9.3036, 0, -104.2536) (-9.45, 0, -101.85) (-9.3036, 0, -99.4464) (0, 0, -99.3)
sketch "krokace_nalezato_dira" plane through (0, 0, -25.0073) normal (0, 0, -1) x (-1, 0, 0)
  line L0 (74.9628, -2) -> (34.9628, -2)
  line L1 (34.9628, -2) -> (34.9628, -17)
  line L2 (34.9628, -17) -> (39.9159, -17)
  line L3 (39.9159, -17) -> (74.9628, -17)
  line L4 (74.9628, -17) -> (74.9628, -2)
  line L5 (47.0372, -41) -> (27.0372, -41)
  line L6 (27.0372, -41) -> (27.0372, -11)
  line L7 (27.0372, -11) -> (47.0372, -11)
  line L8 (47.0372, -11) -> (47.0372, -41)
  line L9 (75.0372, -40) -> (75.0372, 5)
  line L10 (98.5902, 0) -> (15, 0)
  line L11 (0, 1.75) -> (0, 22.5)
  line L12 (-47.0372, -41) -> (-27.0372, -41)
  line L13 (-27.0372, -41) -> (-27.0372, -11)
  line L14 (-27.0372, -11) -> (-47.0372, -11)
  line L15 (-47.0372, -11) -> (-47.0372, -41)
  dimension "d361" = 20
  dimension "d362" = 30
  dimension "d363" = 28
  dimension "d364" = 11
  constraint horizontal L5
  constraint vertical L6
  constraint horizontal L7
  constraint vertical L8
  constraint symmetric L5.start L11 L12.start
  constraint symmetric L5.end L11 L12.end
  constraint symmetric L6.end L11 L13.end
  constraint symmetric L7.end L11 L14.end
  measures "d361" distance of L5.start L5.end
  measures "d362" distance of L5.start L7.end
  measures "d363" distance of L8 L9
  measures "d364" distance of L7 L10
extrude "Extrude39" cut sketch "krokace_nalezato_dira" against normal blind 5 contours L1 L2 L3 L7 L8 | L1 L2 L3 L5 L6 L7 L8 | L12 L13 L14 L15
sketch "dira_rfid_konektor" plane through (0, 0, 0) normal (0, 1, 0) x (1, 0, 0)
  line L0 (32.95, 78.0037) -> (18.95, 78.0037)
  line L1 (17.95, 77.0037) -> (17.95, 54.0037)
  line L2 (18.95, 53.0037) -> (32.95, 53.0037)
  line L3 (33.95, 54.0037) -> (33.95, 77.0037)
  line L4 (-20, 83.0037) -> (20, 83.0037)
  arc A0 (33.95, 77.0037) -> (32.95, 78.0037) centre (32.95, 77.0037) ccw
  arc A1 (18.95, 78.0037) -> (17.95, 77.0037) centre (18.95, 77.0037) ccw
  arc A2 (17.95, 54.0037) -> (18.95, 53.0037) centre (18.95, 54.0037) ccw
  arc A3 (32.95, 53.0037) -> (33.95, 54.0037) centre (32.95, 54.0037) ccw
  line L5 (15, 54) -> (39, 54)
  line L6 (40, 53) -> (40, 41)
  line L7 (39, 40) -> (15, 40)
  line L8 (14, 41) -> (14, 53)
  arc A4 (15, 54) -> (14, 53) centre (15, 53) ccw
  arc A5 (40, 53) -> (39, 54) centre (39, 53) ccw
  arc A6 (39, 40) -> (40, 41) centre (39, 41) ccw
  arc A7 (14, 41) -> (15, 40) centre (15, 41) ccw
  line L9 (16.493, 83.0037) -> (25.7483, 83.0037)
  line L10 (25.7483, 83.0037) -> (25.7483, 76.4305)
  line L11 (25.7483, 76.4305) -> (16.493, 76.4305)
  line L12 (16.493, 76.4305) -> (16.493, 83.0037)
  point P0 (33.95, 78.0037)
  point P1 (17.95, 78.0037)
  point P2 (33.95, 53.0037)
  point P3 (14.95, 57.25)
  dimension "d367" = 3
  dimension "d368" = 16
  dimension "d369" = 25
  dimension "d370" = 5
  dimension "d371" = 1
  dimension "d379" = 1
  constraint horizontal L0
  constraint vertical L1
  constraint horizontal L2
  constraint vertical L3
  constraint coincident P0 L0
  constraint coincident P0 L3
  constraint tangent L0 A0
  constraint tangent L3 A0
  constraint coincident P1 L0
  constraint coincident P1 L1
  constraint tangent L0 A1
  constraint tangent L1 A1
  constraint equal A0 A1
  constraint tangent L1 A2
  constraint tangent L2 A2
  constraint equal A0 A2
  constraint coincident P2 L2
  constraint coincident P2 L3
  constraint tangent L2 A3
  constraint tangent L3 A3
  constraint equal A0 A3
  constraint horizontal L5
  constraint vertical L6
  constraint horizontal L7
  constraint vertical L8
  constraint tangent L5 A4
  constraint tangent L8 A4
  constraint tangent L5 A5
  constraint tangent L6 A5
  constraint equal A4 A5
  constraint tangent L6 A6
  constraint tangent L7 A6
  constraint equal A4 A6
  constraint tangent L7 A7
  constraint tangent L8 A7
  constraint equal A4 A7
  constraint horizontal L9
  constraint vertical L10
  constraint horizontal L11
  constraint vertical L12
  constraint coincident L4 L9.start
  measures "d367" distance of L1 P3
  measures "d368" distance of P0 P1
  measures "d369" distance of P0 P2
  measures "d370" distance of L0 L4
  measures "d371" radius of A0
  measures "d379" radius of A4
extrude "Extrude40" cut sketch "dira_rfid_konektor" along normal blind 5
sketch "sloupky_patro" plane through (0, 0, 0) normal (0, 1, 0) x (1, 0, 0)
  circle A0 centre (30, -94.9953) radius 5
  line L0 (0, 105) -> (0, -105)
  circle A1 centre (30, -94.9953) radius 1.85
  line L1 (-105, 0) -> (104.2756, 0.0073)
  circle A2 centre (29.9934, 95.0047) radius 5
  circle A3 centre (29.9934, 95.0047) radius 1.85
  circle A4 centre (-30, -94.9953) radius 5
  circle A5 centre (-30, -94.9953) radius 1.85
  circle A6 centre (-29.9934, 95.0047) radius 5
  circle A7 centre (-29.9934, 95.0047) radius 1.85
  dimension "d374" = 30
  dimension "d375" = 3.7
  dimension "d376" = 95
  constraint concentric A0 A1
  constraint symmetric A0 L1 A2
  constraint symmetric A1 L1 A3
  constraint symmetric A0 L0 A4
  constraint symmetric L0 A1 A5
  constraint symmetric L0 A2 A6
  constraint symmetric L0 A3 A7
  measures "d374" distance of A0.centre L0
  measures "d375" diameter of A1
  measures "d376" distance of A0.centre L1
extrude "Extrude41" add sketch "sloupky_patro" against normal blind 40